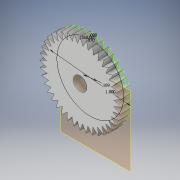
# Autodesk Inventor part: phonegearfinalBIG
Saved by Autodesk Inventor 2018 (Build 220112000, 112)
## iProperties
Created: 2019-03-12
Part Number: phonegearfinalBIG
Material: Generic
Document SubType Name: Modeling
Designer: F8PLTW
Density: 1 g/cm^3
Appearance: Default
Author: F8PLTW
Autodesk Inventor part; units mm, degrees
ref_plane "YZ Plane" through (0, 0, 0) normal (1, 0, 0) x (0, 1, 0)
ref_plane "XZ Plane" through (0, 0, 0) normal (0, 1, 0) x (-1, 0, 0)
ref_plane "XY Plane" through (0, 0, 0) normal (0, 0, 1) x (1, 0, 0)
sketch "Sketch1" plane through (0, 0, 0) normal (0, 0, 1) x (1, 0, 0)
  circle A0 centre (-4.7103, 5.2603) radius 12.7 construction
  line L0 (-4.6585, 14.5504) -> (-4.6585, 17.9602) construction
  line L1 (-5.0163, 15.6864) -> (-5.0163, 15.6864)
  line L2 (-3.7695, 15.6742) -> (-4.6585, 17.9602)
  line L3 (-5.5475, 15.6742) -> (-4.6585, 17.9602)
  line L4 (-5.5475, 15.6742) -> (-3.7695, 15.6742)
  line L5 (-7.1663, 15.415) -> (-6.6459, 17.8119)
  line L6 (-5.4102, 15.6931) -> (-6.6459, 17.8119)
  line L7 (-7.1663, 15.415) -> (-5.4102, 15.6931)
  line L8 (-8.7246, 14.9058) -> (-8.5855, 17.3546)
  line L9 (-7.0336, 15.4552) -> (-8.5855, 17.3546)
  line L10 (-8.7246, 14.9058) -> (-7.0336, 15.4552)
  line L11 (-10.1841, 14.159) -> (-10.4298, 16.5995)
  line L12 (-8.5999, 14.9662) -> (-10.4298, 16.5995)
  line L13 (-10.1841, 14.159) -> (-8.5999, 14.9662)
  line L14 (-11.5088, 13.1932) -> (-12.1332, 15.5651)
  line L15 (-10.0703, 14.2383) -> (-12.1332, 15.5651)
  line L16 (-11.5088, 13.1932) -> (-10.0703, 14.2383)
  line L17 (-12.666, 12.032) -> (-13.6539, 14.2771)
  line L18 (-11.4088, 13.2892) -> (-13.6539, 14.2771)
  line L19 (-12.666, 12.032) -> (-11.4088, 13.2892)
  line L20 (-13.6274, 10.7041) -> (-14.9543, 12.767)
  line L21 (-12.5823, 12.1425) -> (-14.9543, 12.767)
  line L22 (-13.6274, 10.7041) -> (-12.5823, 12.1425)
  line L23 (-14.3692, 9.2421) -> (-16.0025, 11.072)
  line L24 (-13.562, 10.8263) -> (-16.0025, 11.072)
  line L25 (-14.3692, 9.2421) -> (-13.562, 10.8263)
  line L26 (-14.8732, 7.6821) -> (-16.7726, 9.234)
  line L27 (-14.3238, 9.3731) -> (-16.7726, 9.234)
  line L28 (-14.8732, 7.6821) -> (-14.3238, 9.3731)
  line L29 (-15.1269, 6.0624) -> (-17.2457, 7.2981)
  line L30 (-14.8488, 7.8185) -> (-17.2457, 7.2981)
  line L31 (-15.1269, 6.0624) -> (-14.8488, 7.8185)
  line L32 (-15.1242, 4.423) -> (-17.4102, 5.312)
  line L33 (-15.1242, 6.201) -> (-17.4102, 5.312)
  line L34 (-15.1242, 4.423) -> (-15.1242, 6.201)
  line L35 (-14.865, 2.8043) -> (-17.2619, 3.3247)
  line L36 (-15.1431, 4.5604) -> (-17.2619, 3.3247)
  line L37 (-14.865, 2.8043) -> (-15.1431, 4.5604)
  line L38 (-14.3557, 1.2459) -> (-16.8046, 1.385)
  line L39 (-14.9052, 2.9369) -> (-16.8046, 1.385)
  line L40 (-14.3557, 1.2459) -> (-14.9052, 2.9369)
  line L41 (-13.609, -0.2135) -> (-16.0494, -0.4592)
  line L42 (-14.4162, 1.3707) -> (-16.0494, -0.4592)
  line L43 (-13.609, -0.2135) -> (-14.4162, 1.3707)
  line L44 (-12.6432, -1.5382) -> (-15.0151, -2.1627)
  line L45 (-13.6882, -0.0998) -> (-15.0151, -2.1627)
  line L46 (-12.6432, -1.5382) -> (-13.6882, -0.0998)
  line L47 (-11.482, -2.6955) -> (-13.727, -3.6833)
  line L48 (-12.7392, -1.4382) -> (-13.727, -3.6833)
  line L49 (-11.482, -2.6955) -> (-12.7392, -1.4382)
  line L50 (-10.154, -3.6569) -> (-12.2169, -4.9837)
  line L51 (-11.5925, -2.6118) -> (-12.2169, -4.9837)
  line L52 (-10.154, -3.6569) -> (-11.5925, -2.6118)
  line L53 (-8.6921, -4.3987) -> (-10.522, -6.0319)
  line L54 (-10.2763, -3.5915) -> (-10.522, -6.0319)
  line L55 (-8.6921, -4.3987) -> (-10.2763, -3.5915)
  line L56 (-7.1321, -4.9026) -> (-8.684, -6.802)
  line L57 (-8.823, -4.3532) -> (-8.684, -6.802)
  line L58 (-7.1321, -4.9026) -> (-8.823, -4.3532)
  line L59 (-5.5124, -5.1564) -> (-6.7481, -7.2752)
  line L60 (-7.2685, -4.8782) -> (-6.7481, -7.2752)
  line L61 (-5.5124, -5.1564) -> (-7.2685, -4.8782)
  line L62 (-3.873, -5.1536) -> (-4.762, -7.4396)
  line L63 (-5.651, -5.1536) -> (-4.762, -7.4396)
  line L64 (-3.873, -5.1536) -> (-5.651, -5.1536)
  line L65 (-2.2542, -4.8944) -> (-2.7747, -7.2913)
  line L66 (-4.0103, -5.1726) -> (-2.7747, -7.2913)
  line L67 (-2.2542, -4.8944) -> (-4.0103, -5.1726)
  line L68 (-0.6959, -4.3852) -> (-0.835, -6.834)
  line L69 (-2.3869, -4.9346) -> (-0.835, -6.834)
  line L70 (-0.6959, -4.3852) -> (-2.3869, -4.9346)
  line L71 (0.7635, -3.6384) -> (1.0093, -6.0789)
  line L72 (-0.8207, -4.4456) -> (1.0093, -6.0789)
  line L73 (0.7635, -3.6384) -> (-0.8207, -4.4456)
  line L74 (2.0882, -2.6726) -> (2.7127, -5.0446)
  line L75 (0.6498, -3.7177) -> (2.7127, -5.0446)
  line L76 (2.0882, -2.6726) -> (0.6498, -3.7177)
  line L77 (3.2455, -1.5114) -> (4.2333, -3.7565)
  line L78 (1.9883, -2.7686) -> (4.2333, -3.7565)
  line L79 (3.2455, -1.5114) -> (1.9883, -2.7686)
  line L80 (4.2069, -0.1835) -> (5.5337, -2.2464)
  line L81 (3.1618, -1.6219) -> (5.5337, -2.2464)
  line L82 (4.2069, -0.1835) -> (3.1618, -1.6219)
  line L83 (4.9487, 1.2785) -> (6.5819, -0.5514)
  line L84 (4.1415, -0.3057) -> (6.5819, -0.5514)
  line L85 (4.9487, 1.2785) -> (4.1415, -0.3057)
  line L86 (5.4527, 2.8385) -> (7.3521, 1.2866)
  line L87 (4.9032, 1.1475) -> (7.3521, 1.2866)
  line L88 (5.4527, 2.8385) -> (4.9032, 1.1475)
  line L89 (5.7064, 4.4582) -> (7.8252, 3.2225)
  line L90 (5.4282, 2.702) -> (7.8252, 3.2225)
  line L91 (5.7064, 4.4582) -> (5.4282, 2.702)
  line L92 (5.7036, 6.0976) -> (7.9896, 5.2086)
  line L93 (5.7036, 4.3196) -> (7.9896, 5.2086)
  line L94 (5.7036, 6.0976) -> (5.7036, 4.3196)
  line L95 (5.4444, 7.7163) -> (7.8414, 7.1959)
  line L96 (5.7226, 5.9602) -> (7.8414, 7.1959)
  line L97 (5.4444, 7.7163) -> (5.7226, 5.9602)
  line L98 (4.9352, 9.2746) -> (7.384, 9.1356)
  line L99 (5.4846, 7.5837) -> (7.384, 9.1356)
  line L100 (4.9352, 9.2746) -> (5.4846, 7.5837)
  line L101 (4.1885, 10.7341) -> (6.6289, 10.9798)
  line L102 (4.9957, 9.1499) -> (6.6289, 10.9798)
  line L103 (4.1885, 10.7341) -> (4.9957, 9.1499)
  line L104 (3.2226, 12.0588) -> (5.5946, 12.6832)
  line L105 (4.2677, 10.6203) -> (5.5946, 12.6832)
  line L106 (3.2226, 12.0588) -> (4.2677, 10.6203)
  line L107 (2.0614, 13.2161) -> (4.3065, 14.2039)
  line L108 (3.3187, 11.9588) -> (4.3065, 14.2039)
  line L109 (2.0614, 13.2161) -> (3.3187, 11.9588)
  line L110 (0.7335, 14.1774) -> (2.7964, 15.5043)
  line L111 (2.1719, 13.1324) -> (2.7964, 15.5043)
  line L112 (0.7335, 14.1774) -> (2.1719, 13.1324)
  line L113 (-0.7285, 14.9192) -> (1.1015, 16.5525)
  line L114 (0.8557, 14.1121) -> (1.1015, 16.5525)
  line L115 (-0.7285, 14.9192) -> (0.8557, 14.1121)
  line L116 (-2.2885, 15.4232) -> (-0.7366, 17.3226)
  line L117 (-0.5975, 14.8738) -> (-0.7366, 17.3226)
  line L118 (-2.2885, 15.4232) -> (-0.5975, 14.8738)
  line L119 (-3.9081, 15.677) -> (-2.6725, 17.7957)
  line L120 (-2.152, 15.3988) -> (-2.6725, 17.7957)
  line L121 (-3.9081, 15.677) -> (-2.152, 15.3988)
  circle A1 centre (-4.7103, 5.2603) radius 2.15
  circle A2 centre (-4.7103, 5.2603) radius 10.5951
  point P0 (0, 0)
  point P1 (-4.6585, 16.2553)
  dimension "d0" = 25.4
  dimension "d4" = 360
  dimension "d10" = 4.3
  dimension "d13" = 1.778
  dimension "d15" = 2.286
  constraints: 244 end point, 2 centre point, 2 coincident, 2 horizontal, 1 midpoint, 1 symmetric about line, 1 vertical, 244 other
  measures "d10" diameter of A1
  measures "d13" distance of L3.start L2.start
  measures "d15" distance from line of L0.end L4
extrude "Extrusion1" [suppressed]
ref_plane "Work Plane1" through (0, 0, 3) normal (0, 0, 1) x (1, 0, 0)
sketch "Sketch3" plane through (0, 0, 3) normal (0, 0, 1) x (1, 0, 0)
  point P0 (0, 0)
sketch "Sketch4" plane through (0, 0, 3) normal (0, 0, 1) x (1, 0, 0)
  point P0 (0, 0)
extrude "Extrusion4" add sketch "Sketch1" along normal blind 3.175
body "Solid1"
